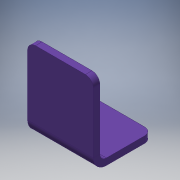
# Autodesk Inventor part: Lamiera 10mm supporto asse
Saved by Autodesk Inventor 2018 (Build 220112000, 112)
## iProperties
Created: 2020-06-03
Part Number: Lamiera 10mm supporto asse
Material: Generico
Document SubType Name: Lamiera
Designer: Francesco
Density: 1 g/cm^3
Sheet Metal Rule: Default_mm
Appearance: Violetto
Author: Francesco
Autodesk Inventor part; units mm, degrees
ref_plane "YZ Plane" through (0, 0, 0) normal (1, 0, 0) x (0, 1, 0)
ref_plane "XZ Plane" through (0, 0, 0) normal (0, 1, 0) x (-1, 0, 0)
ref_plane "XY Plane" through (0, 0, 0) normal (0, 0, 1) x (1, 0, 0)
sketch "Schizzo1" plane through (0, 0, 0) normal (0, 0, 1) x (1, 0, 0)
  line L0 (-25, 17.5) -> (25, 17.5)
  line L1 (25, 17.5) -> (25, -17.5)
  line L2 (25, -17.5) -> (-25, -17.5)
  line L3 (-25, -17.5) -> (-25, 17.5)
  line L4 (-25, 17.5) -> (25, -17.5) construction
  line L5 (25, 17.5) -> (-25, -17.5) construction
  point P0 (0, 0)
  dimension "d0" = 50
  dimension "d1" = 35
  measures "d0" distance of L1.end L2.end
  measures "d1" distance of L0.end L1.end
extrude "Piano1" add sketch "Schizzo1" along normal blind 5
sketch "Schizzo2" plane through (25, -22.5, 10) normal (0, -1, 0) x (1, 0, 0)
  line L0 (-50, 0) -> (0, 0)
  line L1 (0, 0) -> (0, 52)
  line L2 (0, 52) -> (-50, 52)
  line L3 (-50, 52) -> (-50, 0)
  constraints: 6 end point, 1 horizontal, 1 perpendicular, 1 vertical
edge flange "Flangia1" height 62 angle 90 thickness 5 bend radius 5 thickness toward (0, -1, 0) relief tear relief width 5 relief depth 2.5 edges at (0, -17.5, 5) wall of the first edge with corners at (-25, -22.5, 10) (25, -22.5, 10) (25, -22.5, 62) (-25, -22.5, 62)
bend "Piega (Bend)1"
corner "Angolo1"
fillet "Arrotondamento angolo1" radius 6 4 edges at (-25, 17.5, 2.5) (25, 17.5, 2.5) (25, -25, 62) (-25, -25, 62)
equation "\"d2\" = Spessore"
equation "\"d3\" = LarghezzaScaricoPiega"
equation "\"d4\" = ProfonditàScaricoPiega"
equation "\"d5\" = ResiduoMinimo"
equation "\"d6\" = RaggioTransizione"
equation "\"d9\" = RaggioPiega"
equation "\"d10\" = DimensioniScaricoAngolo"
equation "\"d11\" = DimensioneGioco"
equation "\"d12\" = Dimensione_raggio_Jacobi"
equation "\"RaggioPiega\" = Spessore"
equation "\"LarghezzaScaricoPiega\" = Spessore"
equation "\"ProfonditàScaricoPiega\" = 0.5 * Spessore"
equation "\"RaggioTransizione\" = RaggioPiega"
equation "\"Dimensione_raggio_Jacobi\" = RaggioPiega"
equation "\"DimensioneGioco\" = Spessore"
equation "\"Spessore\" = 5"
equation "\"ResiduoMinimo\" = 10"
equation "\"DimensioniScaricoAngolo\" = 20"
